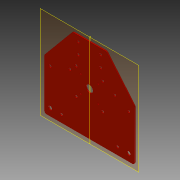
# Autodesk Inventor part: SM-S01
Saved by Autodesk Inventor 2013 (Build 170138000, 138)
## iProperties
Company: ShapeOko.com
Created: 2011-08-17
Part Number: SM-S01
Material: Steel, Mild
Document SubType Name: Modeling
Designer: ERF
Mass: 305.957 g
Surface Area: 426.739 cm^2
Volume: 38.9259 cm^3
Density: 7.86 g/cm^3
Project: Shapeoko
Checked By: ERF
Catalog Web Link: www.shapeoko.com/purchase
Description: motor mount plate
Vendor: Shapeoko
Stock Number: SM-S01
Title: Mounting Plate
Subject: Structure
Author: ERF
Autodesk Inventor part; units mm, degrees
ref_plane "YZ Plane" through (0, 0, 0) normal (1, 0, 0) x (0, 1, 0)
ref_plane "XZ Plane" through (0, 0, 0) normal (0, 1, 0) x (-1, 0, 0)
ref_plane "XY Plane" through (0, 0, 0) normal (0, 0, 1) x (1, 0, 0)
sketch "Sketch1" plane through (0, 0, 0) normal (0, 0, 1) x (1, 0, 0)
  line L0 (10.9384, 8.2044) -> (170.9384, 8.2044)
  line L1 (170.9384, 8.2044) -> (170.9384, 98.2044)
  line L2 (10.9384, 98.2044) -> (10.9384, 8.2044)
  line L3 (10.9384, 98.2044) -> (60.9384, 158.2044)
  line L4 (60.9384, 158.2044) -> (120.9384, 158.2044)
  line L5 (120.9384, 158.2044) -> (170.9384, 98.2044)
  dimension "d0" = 160
  dimension "d4" = 60
  dimension "d5" = 50
  dimension "d6" = 90
  dimension "d7" = 90
  dimension "d8" = 150
  constraints: 12 end point, 2 perpendicular, 1 horizontal, 1 parallel
  measures "d0" distance of L0.start L0.end
  measures "d4" distance of L3.end L4.end
  measures "d5" horizontal distance of L1.end L4.end
  measures "d6" distance of L0.end L1.end
  measures "d7" distance of L0.start L2.start
  measures "d8" distance between parallel lines of L0 L4
extrude "Extrusion1" add sketch "Sketch1" along normal blind 1.8974
sketch "Sketch2" plane through (0, 0, 1.8974) normal (0, 0, 1) x (1, 0, 0)
  line L0 (10.9384, 8.2044) -> (10.9384, 98.2044) projected
  line L1 (170.9384, 8.2044) -> (10.9384, 8.2044) projected
  circle A0 centre (20.9384, 20.9044) radius 3.5685
  circle A1 centre (20.9384, 85.5044) radius 2.5
  dimension "d11" = 7.137
  dimension "d12" = 12.7
  dimension "d13" = 10
  dimension "d14" = 10
  dimension "d15" = 64.6
  dimension "d16" = 5
  constraints: 2 centre point
  measures "d11" diameter of A0
  measures "d12" distance from line of L1 A0.centre
  measures "d13" distance from line of L0 A0.centre
  measures "d14" distance from line of L0 A1.centre
  measures "d15" distance of A0.centre A1.centre
  measures "d16" diameter of A1
extrude "Extrusion2" cut sketch "Sketch2" against normal through all
pattern_linear "Rectangular Pattern1" count 2 spacing 140 along (1, 0, 0) of "Extrusion2"
sketch "Sketch3" plane through (0, 0, 1.8974) normal (0, 0, 1) x (1, 0, 0)
  line L0 (10.9384, 8.2044) -> (10.9384, 98.2044) projected
  line L1 (170.9384, 8.2044) -> (10.9384, 8.2044) projected
  circle A0 centre (90.9384, 85.5044) radius 6.5
  circle A1 centre (75.4444, 70.0104) radius 1.5
  circle A2 centre (106.4324, 70.0104) radius 1.5
  circle A3 centre (75.4444, 100.9984) radius 1.5
  circle A4 centre (106.4324, 100.9984) radius 1.5
  dimension "d22" = 13
  dimension "d23" = 80
  dimension "d24" = 77.3
  dimension "d27" = 3
  dimension "d28" = 61.806
  dimension "d29" = 64.506
  dimension "d30" = 3
  dimension "d31" = 61.806
  dimension "d32" = 95.494
  dimension "d33" = 3
  dimension "d34" = 3
  dimension "d35" = 64.506
  dimension "d36" = 92.794
  dimension "d37" = 92.794
  dimension "d38" = 95.494
  constraints: 5 centre point
  measures "d22" diameter of A0
  measures "d23" distance from line of L0 A0.centre
  measures "d24" distance from line of L1 A0.centre
  measures "d27" diameter of A1
  measures "d28" distance from line of L1 A1.centre
  measures "d29" distance from line of L0 A1.centre
  measures "d30" diameter of A2
  measures "d31" distance from line of L1 A2.centre
  measures "d32" distance from line of L0 A2.centre
  measures "d33" diameter of A3
  measures "d34" diameter of A4
  measures "d35" distance from line of L0 A3.centre
  measures "d36" distance from line of L1 A3.centre
  measures "d37" distance from line of L1 A4.centre
  measures "d38" distance from line of L0 A4.centre
extrude "Extrusion3" cut sketch "Sketch3" against normal through all
sketch "Sketch4" plane through (0, 0, 1.8974) normal (0, 0, 1) x (1, 0, 0)
  circle A0 centre (160.9384, 85.5044) radius 2.5 projected
  circle A1 centre (20.9384, 85.5044) radius 2.5 projected
  line L0 (10.9384, 8.2044) -> (10.9384, 98.2044) projected
  line L1 (170.9384, 98.2044) -> (170.9384, 8.2044) projected
  circle A2 centre (55.9384, 98.2044) radius 2.5
  circle A3 centre (135.9384, 98.2044) radius 2.5
  dimension "d39" = 45
  dimension "d40" = 12.7
  dimension "d41" = 5
  dimension "d42" = 35
  dimension "d43" = 12.7
  dimension "d44" = 5
  constraints: 2 centre point
  measures "d39" distance from line of L0 A2.centre
  measures "d40" vertical distance of A1.centre A2.centre
  measures "d41" diameter of A2
  measures "d42" distance from line of L1 A3.centre
  measures "d43" vertical distance of A0.centre A3.centre
  measures "d44" diameter of A3
extrude "Extrusion4" cut sketch "Sketch4" against normal through all contours A2 | A3
sketch "Sketch5" plane through (0, 0, 1.8974) normal (0, 0, 1) x (1, 0, 0)
  line L0 (60.9384, 158.2044) -> (120.9384, 158.2044) projected
  circle A0 centre (110.9384, 148.2044) radius 2.5
  circle A1 centre (110.9384, 128.2044) radius 2.5
  dimension "d47" = 10
  dimension "d48" = 10
  dimension "d49" = 20
  dimension "d50" = 10
  dimension "d51" = 5
  dimension "d52" = 5
  constraints: 2 centre point
  measures "d47" distance from line of L0 A0.centre
  measures "d48" horizontal distance of L0.end A0.centre
  measures "d49" distance of A0.centre A1.centre
  measures "d50" horizontal distance of L0.end A1.centre
  measures "d51" diameter of A0
  measures "d52" diameter of A1
extrude "Extrusion5" cut sketch "Sketch5" against normal through all
sketch "Sketch6" plane through (0, 0, 1.8974) normal (0, 0, 1) x (1, 0, 0)
  line L0 (10.9384, 8.2044) -> (10.9384, 98.2044) projected
  line L1 (170.9384, 8.2044) -> (10.9384, 8.2044) projected
  circle A0 centre (67.3264, 61.8746) radius 2.54
  dimension "d55" = 56.388
  dimension "d56" = 53.6702
  dimension "d57" = 5.08
  constraints: 1 centre point
  measures "d55" distance from line of L0 A0.centre
  measures "d56" distance from line of L1 A0.centre
  measures "d57" diameter of A0
extrude "Extrusion6" cut sketch "Sketch6" against normal through all
pattern_linear "Rectangular Pattern2" count 2 spacing 47.244 along (1, 0, 0) count 2 spacing 47.244 along (0, 1, 0) of "Extrusion6"
fillet "Fillet2" radius 3.175 6 edges at (120.9384, 158.2044, 0.9487) (60.9384, 158.2044, 0.9487) (170.9384, 98.2044, 0.9487) (170.9384, 8.2044, 0.9487) (10.9384, 98.2044, 0.9487) (10.9384, 8.2044, 0.9487)
sketch "Sketch7" plane through (0, 0, 0) normal (0, 0, -1) x (-1, 0, 0)
  line L0 (-10.9384, 97.0549) -> (-10.9384, 11.3794) projected
  line L1 (-170.9384, 11.3794) -> (-170.9384, 97.0549) projected
  line L2 (-14.1134, 8.2044) -> (-167.7634, 8.2044) projected
  circle A0 centre (-140.9384, 20.9044) radius 2.5
  circle A1 centre (-40.9384, 20.9044) radius 2.5
  dimension "d68" = 5
  dimension "d69" = 12.7
  dimension "d70" = 30
  dimension "d71" = 5
  dimension "d72" = 30
  dimension "d73" = 12.7
  constraints: 2 centre point
  measures "d68" diameter of A0
  measures "d69" distance from line of L2 A0.centre
  measures "d70" distance from line of L1 A0.centre
  measures "d71" diameter of A1
  measures "d72" distance from line of L0 A1.centre
  measures "d73" distance from line of L2 A1.centre
extrude "Extrusion7" cut sketch "Sketch7" against normal through all
ref_plane "Work Plane1" through (90.9384, 158.2044, 1.8974) normal (0, 0, 1) x (1, 0, 0)
ref_plane "Work Plane2" through (90.9384, 158.2044, 1.8974) normal (-1, 0, 0) x (0, 0, 1)
mirror "Mirror1" about plane through (90.9384, 158.2044, 1.8974) normal (-1, 0, 0) of "Extrusion5"
equation "\"d7\" = d6"
equation "\"d30\" = d27"
equation "\"d31\" = d28"
equation "\"d33\" = d27"
equation "\"d34\" = d27"
equation "\"d35\" = d29"
equation "\"d50\" = d48"
body "Solid1"
